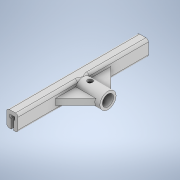
# Autodesk Inventor part: wiper
Saved by Autodesk Inventor 2021 (Build 250183000, 183)
## iProperties
Created: 2021-04-19
Part Number: wiper
Material: 일반
Document SubType Name: Modeling
Designer: Dongyoon
Density: 1 g/cm^3
Appearance: 기본값
Author: Dongyoon
Autodesk Inventor part; units mm, degrees
ref_plane "YZ Plane" through (0, 0, 0) normal (1, 0, 0) x (0, 1, 0)
ref_plane "XZ Plane" through (0, 0, 0) normal (0, 1, 0) x (-1, 0, 0)
ref_plane "XY Plane" through (0, 0, 0) normal (0, 0, 1) x (1, 0, 0)
sketch "스케치1" plane through (0, 0, 0) normal (1, 0, 0) x (0, 1, 0)
  line L0 (-6.5, -52.5) -> (6.5, -52.5)
  line L1 (6.5, -52.5) -> (6.5, 52.5)
  line L2 (6.5, 52.5) -> (-6.5, 52.5)
  line L3 (-6.5, 52.5) -> (-6.5, -52.5)
  line L4 (-6.5, -52.5) -> (6.5, 52.5) construction
  line L5 (6.5, -52.5) -> (-6.5, 52.5) construction
  point P0 (0, 0)
  dimension "d0" = 13
  dimension "d1" = 105
  constraints: 12 end point, 2 midpoint, 2 parallel, 1 horizontal, 1 perpendicular
  measures "d0" distance of L1.end L2.end
  measures "d1" distance of L0.end L1.end
extrude "돌출1" add sketch "스케치1" along normal blind 9
sketch "스케치2" plane through (0, -6.5, 52.5) normal (0, 0, 1) x (1, 0, 0)
  line L0 (2.5, 10) -> (6.5, 10)
  line L1 (6.5, 10) -> (6.5, 7.4)
  line L2 (6.5, 7.4) -> (5.6, 7.4)
  line L3 (5.6, 7.4) -> (5.5, 0)
  line L4 (0, 0) -> (9, 0) projected
  line L5 (3.5, 0) -> (3.4, 7.4)
  line L6 (3.4, 7.4) -> (2.5, 7.4)
  line L7 (2.5, 7.4) -> (2.5, 10)
  line L8 (5.5, 0) -> (3.5, 0)
  line L9 (9, 13) -> (9, 0) projected
  line L10 (0, 13) -> (9, 13) projected
  point P0 (0, 6.5)
  dimension "d4" = 4
  dimension "d6" = 2.5
  dimension "d7" = 2.6
  dimension "d8" = 2.6
  dimension "d9" = 3
  dimension "d10" = 2.2
  dimension "d11" = 0.9
  dimension "d12" = 2
  dimension "d13" = 3.5
  constraints: 16 end point, 4 perpendicular, 2 point on line, 1 collinear, 1 horizontal
  measures "d4" distance of L0.start L0.end
  measures "d6" distance between parallel lines of L9 L1
  measures "d7" distance of L0.end L1.end
  measures "d8" distance of L6.end L0.start
  measures "d9" distance between parallel lines of L10 L0
  measures "d10" distance of L2.end L5.end
  measures "d11" distance of L5.end L6.end
  measures "d12" distance of L3.end L5.start
  measures "d13" distance of L4.end L3.end
extrude "돌출2" cut sketch "스케치2" against normal through all
sketch "스케치3" plane through (9, 0, 0) normal (1, 0, 0) x (0, 0, -1)
  circle A0 centre (0, 0) radius 4.5
  circle A1 centre (0, 0) radius 6.5
  dimension "d16" = 9
  constraints: 2 centre point, 2 coincident
  measures "d16" diameter of A0
extrude "돌출3" add sketch "스케치3" along normal blind 20
sketch "스케치4" plane through (0, 0, 0) normal (0, 1, 0) x (-1, 0, 0)
  line L0 (-9, 6.5) -> (-29, 6.5) projected
  line L1 (-24.1828, 7.1664) -> (-10.2269, 21.1223)
  line L2 (-9, 52.5) -> (-9, 0) projected
  point P0 (0, 0)
  dimension "d19" = 45
  constraints: 2 end point
  measures "d19" angle of L0 L1
extrude "리브1" add sketch "스케치4" along normal mid plane 5 rib yes fills toward (-17.1695, 14.109) open curves L1
mirror "미러1" about plane through (0, 0, 0) normal (0, 0, 1) of "리브1"
sketch "스케치5" plane through (0, 0, 0) normal (0, 1, 0) x (-1, 0, 0)
  circle A0 centre (-14.7, 0) radius 2
  line L0 (-9, -52.5) -> (-9, 0) projected
  point P0 (0, 0)
  dimension "d26" = 4
  dimension "d27" = 5.7
  constraints: 1 centre point
  measures "d26" diameter of A0
  measures "d27" distance from line of A0.centre L0
extrude "돌출4" cut sketch "스케치5" along normal blind 20 and the other way blind 10
fillet "모깎기1" radius 2 6 edges at (0, 6.5, 0) (9, 6.5, 26.25) (9, 6.5, -26.25) (9, -6.5, 26.25) (9, -6.5, -26.25) (0, -6.5, 0)
